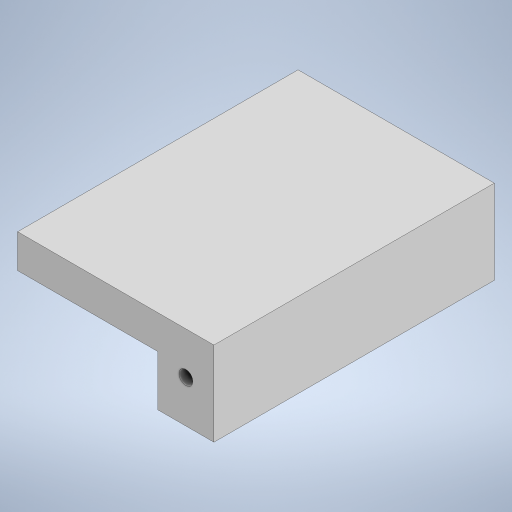
# Autodesk Inventor part: Touchscreen mount L v05
Saved by Autodesk Inventor 2023 (Build 270158000, 158)
## iProperties
Created: 2024-06-29
Part Number: Touchscreen mount L v05
Material: Generic
Document SubType Name: Modeling
Designer: Akramilab
Density: 1 g/cm^3
Appearance: Default
Author: Akramilab
Autodesk Inventor part; units mm, degrees
ref_plane "YZ Plane" through (0, 0, 0) normal (1, 0, 0) x (0, 1, 0)
ref_plane "XZ Plane" through (0, 0, 0) normal (0, 1, 0) x (-1, 0, 0)
ref_plane "XY Plane" through (0, 0, 0) normal (0, 0, 1) x (1, 0, 0)
sketch "Sketch1" plane through (0, 0, 0) normal (0, 0, 1) x (1, 0, 0)
  line L0 (0, 30) -> (20, 30)
  line L1 (20, 30) -> (20, 0)
  line L2 (20, 0) -> (0, 0)
  line L3 (0, 0) -> (0, 30)
  circle A0 centre (10, 15) radius 2.5
  dimension "d0" = 30
  dimension "d1" = 20
  dimension "d5" = 10
  dimension "d6" = 15
  dimension "d7" = 5
  constraints: 8 end point, 2 parallel, 1 centre point, 1 coincident, 1 horizontal, 1 perpendicular
  measures "d0" distance between parallel lines of L2 L0
  measures "d1" distance between parallel lines of L1 L3
  measures "d5" distance from line of point (10, 15) L3
  measures "d6" distance from line of L2 point (10, 15)
  measures "d7" diameter of A0
extrude "Extrusion2" add sketch "Sketch1" along normal blind 25
sketch "Sketch5" plane through (0, 0, 0) normal (0, 0, -1) x (-1, 0, 0)
  line L0 (0, 0) -> (-20, 0) projected
  line L1 (-20, 0) -> (-20, 30) projected
  line L2 (0, 0) -> (-20, 0)
  line L3 (-20, 0) -> (-20, 30)
  line L4 (-20, 30) -> (0, 30)
  line L5 (0, 30) -> (0, 0)
  circle A0 centre (-10, 15) radius 2.5 projected
  circle A1 centre (-10, 15) radius 4.5
  dimension "d17" = 9
  constraints: 8 end point, 2 parallel, 1 centre point, 1 coincident, 1 horizontal, 1 perpendicular
  measures "d17" diameter of A1
extrude "Extrusion5" add sketch "Sketch5" along normal blind 75 contours L0 L1 L4 L5
sketch "Sketch7" plane through (0, 0, -75) normal (0, 0, -1) x (-1, 0, 0)
  line L0 (-20, 30) -> (0, 30) projected
  line L1 (0, 30) -> (50, 30)
  line L2 (50, 30) -> (50, 18)
  line L3 (50, 18) -> (0, 18)
  line L4 (0, 18) -> (0, 30)
  point P0 (0, 0)
  dimension "d25" = 50
  dimension "d26" = 12
  constraints: 8 end point, 2 parallel, 1 horizontal, 1 perpendicular
  measures "d25" distance of L2.end L3.end
  measures "d26" distance of L1.end L2.end
extrude "Extrusion7" add sketch "Sketch7" against normal blind 100
equation "\"d5\" = 0.5 * d1"
equation "\"d6\" = 0.5 * d0"
body "Solid2"
